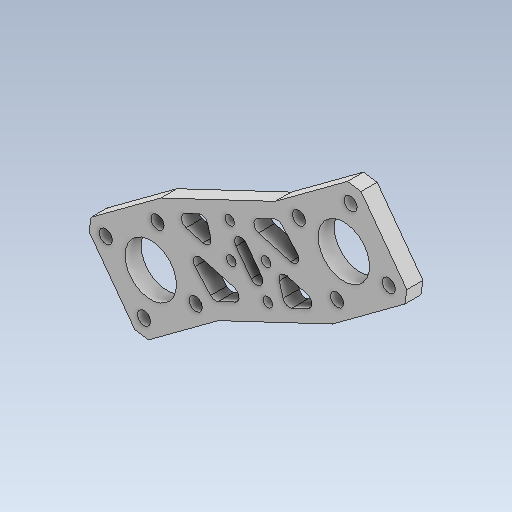
# Autodesk Inventor part: motor_holder_5
Saved by Autodesk Inventor 2020 (Build 240168000, 168)
## iProperties
Created: 2020-05-09
Part Number: motor_holder_5
Material: Generic
Document SubType Name: Modeling
Designer: psrobotics
Density: 1 g/cm^3
Appearance: Default
Author: psrobotics
Autodesk Inventor part; units mm, degrees
ref_plane "YZ Plane" through (0, 0, 0) normal (1, 0, 0) x (0, 1, 0)
ref_plane "XZ Plane" through (0, 0, 0) normal (0, 1, 0) x (-1, 0, 0)
ref_plane "XY Plane" through (0, 0, 0) normal (0, 0, 1) x (1, 0, 0)
sketch "Sketch1" plane through (0, 0, 0) normal (0, 0, 1) x (1, 0, 0)
  line L0 (79.7735, 25.7797) -> (84.0795, 21.6015) projected
  arc A0 (79.9013, 17.2954) -> (84.0795, 21.6015) centre (81.9904, 19.4484) ccw projected
  line L1 (79.9013, 17.2954) -> (75.5952, 21.4737) projected
  arc A1 (79.7735, 25.7797) -> (75.5952, 21.4737) centre (77.6844, 23.6267) ccw projected
  arc A2 (67.2283, 9.1476) -> (72.5711, 11.878) centre (69.8997, 10.5128) ccw projected
  line L2 (67.2283, 9.1476) -> (64.4979, 14.4903) projected
  arc A3 (69.8406, 17.2207) -> (64.4979, 14.4903) centre (67.1692, 15.8555) ccw projected
  line L3 (69.8406, 17.2207) -> (72.5711, 11.878) projected
  circle A4 centre (74.8858, 2.9538) radius 2.075 projected
  circle A5 centre (87.7531, 12.4634) radius 2.075 projected
  circle A6 centre (97.4816, -67.9698) radius 1.5 projected
  circle A7 centre (150.7021, -18.086) radius 1.5 projected
  circle A8 centre (148.9214, -29.9532) radius 1.5 projected
  circle A9 centre (85.6144, -66.1891) radius 1.5 projected
  arc A10 (80.4821, -2.1431) -> (77.7938, -6.6113) centre (99.1499, -16.4177) ccw projected
  arc A11 (83.0041, -2.3614) -> (80.4821, -2.1431) centre (81.6737, -3.0542) ccw projected
  line L4 (85.542, -7.2347) -> (83.0041, -2.3614) projected
  arc A12 (84.6624, -8.6966) -> (85.542, -7.2347) centre (84.655, -7.6966) ccw projected
  line L5 (79.168, -8.7372) -> (84.6624, -8.6966) projected
  arc A13 (77.7938, -6.6113) -> (79.168, -8.7372) centre (79.1569, -7.2373) ccw projected
  arc A14 (113.6374, -24.1387) -> (112.7579, -25.6006) centre (113.6448, -25.1387) ccw projected
  line L6 (119.1319, -24.0981) -> (113.6374, -24.1387) projected
  arc A15 (120.5061, -26.224) -> (119.1319, -24.0981) centre (119.1429, -25.5981) ccw projected
  arc A16 (117.8177, -30.6922) -> (120.5061, -26.224) centre (99.1499, -16.4177) ccw projected
  arc A17 (115.2958, -30.4739) -> (117.8177, -30.6922) centre (116.6262, -29.7811) ccw projected
  line L7 (112.7579, -25.6006) -> (115.2958, -30.4739) projected
  arc A18 (85.0937, -32.5635) -> (84.8754, -35.0855) centre (85.7865, -33.8939) ccw projected
  line L8 (89.967, -30.0256) -> (85.0937, -32.5635) projected
  arc A19 (91.4289, -30.9052) -> (89.967, -30.0256) centre (90.4289, -30.9125) ccw projected
  line L9 (91.4695, -36.3996) -> (91.4289, -30.9052) projected
  arc A20 (89.3436, -37.7738) -> (91.4695, -36.3996) centre (89.9695, -36.4107) ccw projected
  arc A21 (84.8754, -35.0855) -> (89.3436, -37.7738) centre (99.1499, -16.4177) ccw projected
  arc A22 (77.7938, -17.8952) -> (75.8562, -19.5241) centre (77.343, -19.3258) ccw projected
  line L10 (83.0344, -19.5466) -> (77.7938, -17.8952) projected
  arc A23 (83.4461, -21.2023) -> (83.0344, -19.5466) centre (82.7338, -20.5004) ccw projected
  line L11 (79.5897, -25.1161) -> (83.4461, -21.2023) projected
  arc A24 (77.1147, -24.5846) -> (79.5897, -25.1161) centre (78.5212, -24.0633) ccw projected
  arc A25 (75.8562, -19.5241) -> (77.1147, -24.5846) centre (99.1499, -16.4177) ccw projected
  arc A26 (122.4437, -13.3112) -> (121.1852, -8.2507) centre (99.1499, -16.4177) ccw projected
  arc A27 (120.506, -14.9401) -> (122.4437, -13.3112) centre (120.9569, -13.5095) ccw projected
  line L12 (115.2655, -13.2887) -> (120.506, -14.9401) projected
  arc A28 (114.8538, -11.6331) -> (115.2655, -13.2887) centre (115.5661, -12.3349) ccw projected
  line L13 (118.7102, -7.7192) -> (114.8538, -11.6331) projected
  arc A29 (121.1852, -8.2507) -> (118.7102, -7.7192) centre (119.7787, -8.772) ccw projected
  arc A30 (103.9345, -32.1215) -> (102.2789, -32.5332) centre (103.2327, -32.8338) ccw projected
  line L14 (107.8484, -35.9779) -> (103.9345, -32.1215) projected
  arc A31 (107.3169, -38.4529) -> (107.8484, -35.9779) centre (106.7956, -37.0464) ccw projected
  arc A32 (102.2564, -39.7114) -> (107.3169, -38.4529) centre (99.1499, -16.4177) ccw projected
  arc A33 (100.6275, -37.7738) -> (102.2564, -39.7114) centre (102.0581, -38.2246) ccw projected
  line L15 (102.2789, -32.5332) -> (100.6275, -37.7738) projected
  arc A34 (113.4245, 2.2501) -> (108.9563, 4.9385) centre (99.1499, -16.4177) ccw projected
  arc A35 (113.2062, -0.2718) -> (113.4245, 2.2501) centre (112.5134, 1.0586) ccw projected
  line L16 (108.3329, -2.8097) -> (113.2062, -0.2718) projected
  arc A36 (106.871, -1.9302) -> (108.3329, -2.8097) centre (107.871, -1.9228) ccw projected
  line L17 (106.8304, 3.5643) -> (106.871, -1.9302) projected
  arc A37 (108.9563, 4.9385) -> (106.8304, 3.5643) centre (108.3303, 3.5754) ccw projected
  line L18 (90.4515, 3.1426) -> (94.3653, -0.7138) projected
  arc A38 (90.983, 5.6176) -> (90.4515, 3.1426) centre (91.5043, 4.2111) ccw projected
  arc A39 (96.0435, 6.8761) -> (90.983, 5.6176) centre (99.1499, -16.4177) ccw projected
  arc A40 (97.6724, 4.9384) -> (96.0435, 6.8761) centre (96.2417, 5.3893) ccw projected
  line L19 (96.021, -0.3021) -> (97.6724, 4.9384) projected
  arc A41 (94.3653, -0.7138) -> (96.021, -0.3021) centre (95.0672, -0.0015) ccw projected
  circle A42 centre (111.213, -7.5024) radius 1.5 projected
  circle A43 centre (96.7757, -32.2405) radius 2 projected
  circle A44 centre (87.0868, -25.3329) radius 1.5 projected
  circle A45 centre (114.9728, -18.7919) radius 2 projected
  circle A46 centre (101.5242, -0.5948) radius 2 projected
  circle A47 centre (83.3271, -14.0434) radius 2 projected
  circle A48 centre (108.0652, -28.4808) radius 1.5 projected
  circle A49 centre (90.2347, -4.3545) radius 1.5 projected
  circle A50 centre (99.1499, -16.4177) radius 12 projected
  circle A51 centre (57.8427, 39.4747) radius 8 projected
  arc A52 (125.5376, -7.0532) -> (105.1801, 10.9253) centre (99.1499, -16.4177) ccw projected
  line L20 (105.1801, 10.9253) -> (80.5607, 34.8141) projected
  line L21 (80.5607, 34.8141) -> (61.3926, 60.7502) projected
  line L22 (36.4622, 42.3254) -> (61.3926, 60.7502) projected
  line L23 (36.4622, 42.3254) -> (55.6303, 16.3893) projected
  line L24 (55.6303, 16.3893) -> (71.2413, -14.1572) projected
  arc A53 (71.2413, -14.1572) -> (82.4532, -38.8947) centre (99.1499, -16.4177) ccw projected
  arc A54 (84.8089, -44.6016) -> (82.4532, -38.8947) centre (78.8753, -43.7112) ccw projected
  line L25 (84.8089, -44.6016) -> (81.0991, -69.3248) projected
  line L26 (81.0991, -69.3248) -> (100.8777, -72.2926) projected
  line L27 (100.8777, -72.2926) -> (104.5875, -47.5694) projected
  arc A55 (108.5144, -42.8053) -> (104.5875, -47.5694) centre (110.521, -48.4598) ccw projected
  arc A56 (108.5144, -42.8053) -> (121.627, -33.1144) centre (99.1499, -16.4177) ccw projected
  arc A57 (127.3339, -30.7587) -> (121.627, -33.1144) centre (126.4435, -36.6923) ccw projected
  line L28 (127.3339, -30.7587) -> (152.0571, -34.4685) projected
  line L29 (152.0571, -34.4685) -> (155.0249, -14.6899) projected
  line L30 (155.0249, -14.6899) -> (130.3017, -10.9801) projected
  arc A58 (125.5376, -7.0532) -> (130.3017, -10.9801) centre (131.1921, -5.0465) ccw projected
  line L31 (57.8427, 39.4747) -> (99.1499, -16.4177)
  line L32 (57.8427, 39.4747) -> (1.9503, -1.8326)
  line L33 (-1.5997, -23.1081) -> (-19.4302, 1.0181)
  line L34 (-19.4302, 1.0181) -> (61.3926, 60.7502)
  line L35 (61.3926, 60.7502) -> (79.2231, 36.624)
  line L36 (79.2231, 36.624) -> (-1.5997, -23.1081)
  line L37 (-1.5997, -23.1081) -> (61.3926, 60.7502) construction
  line L38 (-19.4302, 1.0181) -> (79.2231, 36.624) construction
  circle A59 centre (55.7441, 25.4892) radius 1.5 projected
  circle A60 centre (59.9412, 53.4603) radius 1.5 projected
  circle A61 centre (71.8282, 37.3762) radius 1.5 projected
  circle A62 centre (43.8571, 41.5733) radius 1.5 projected
  point P0 (0, 0)
  point P1 (29.8965, 18.8211)
  dimension "d0" = 69.5
  dimension "d1" = 30
  dimension "d2" = 100.5
  constraints: 16 end point, 3 midpoint, 3 perpendicular, 2 parallel
  measures "d0" distance of L31.start L32.end
  measures "d1" distance of L33.start L33.end
  measures "d2" distance of L33.end L34.end
extrude "Extrusion1" add sketch "Sketch1" along normal blind 5 contours L36 L23 L32 A51 L31 | L31 A51 L32 L23 L22 L21 L36 | L31 L32 A51 | A51 L32 L31 | L36 L33 L34 L23 | A59 | A60 | A61 | A62
sketch "Sketch2" plane through (0, 0, 5) normal (0, 0, 1) x (1, 0, 0)
  circle A0 centre (57.8427, 39.4747) radius 8 projected
  circle A1 centre (57.8427, 39.4747) radius 8
  point P0 (0, 0)
  dimension "d5" = 16
  constraints: 1 centre point, 1 coincident
  measures "d5" diameter of A1
extrude "Extrusion2" cut sketch "Sketch2" against normal blind 5
sketch "Sketch3" plane through (0, 0, 5) normal (0, 0, 1) x (1, 0, 0)
  circle A0 centre (57.8427, 39.4747) radius 8 projected
  line L0 (79.2231, 36.624) -> (61.3926, 60.7502) projected
  line L1 (61.3926, 60.7502) -> (-19.4302, 1.0181) projected
  line L2 (-19.4302, 1.0181) -> (-1.5997, -23.1081) projected
  line L3 (-1.5997, -23.1081) -> (79.2231, 36.624) projected
  line L4 (43.8571, 41.5733) -> (55.7441, 25.4892)
  line L5 (55.7441, 25.4892) -> (71.8282, 37.3762)
  line L6 (71.8282, 37.3762) -> (59.9412, 53.4603)
  line L7 (59.9412, 53.4603) -> (43.8571, 41.5733)
  line L8 (43.8571, 41.5733) -> (71.8282, 37.3762) construction
  line L9 (55.7441, 25.4892) -> (59.9412, 53.4603) construction
  point P0 (0, 0)
  dimension "d8" = 20
  dimension "d9" = 20
  constraints: 12 end point, 3 parallel, 2 midpoint, 1 perpendicular
  measures "d8" distance of L4.start L4.end
  measures "d9" distance of L5.end L4.end
hole "Hole1" at (43.8571, 41.5733, 5) at (59.9412, 53.4603, 5) at (71.8282, 37.3762, 5) at (55.7441, 25.4892, 5) direction (0, 0, -1) diameter 3 depth 17
sketch "Sketch10" plane through (0, 0, 5) normal (0, 0, 1) x (1, 0, 0)
  circle A0 centre (71.8282, 37.3762) radius 1.5 projected
  circle A1 centre (43.8571, 41.5733) radius 1.5 projected
  circle A2 centre (59.9412, 53.4603) radius 1.5 projected
  circle A3 centre (55.7441, 25.4892) radius 1.5 projected
  circle A4 centre (57.8427, 39.4747) radius 8 projected
  line L0 (-1.5997, -23.1081) -> (79.2231, 36.624) projected
  line L1 (79.2231, 36.624) -> (61.3926, 60.7502) projected
  line L2 (61.3926, 60.7502) -> (-19.4302, 1.0181) projected
  line L3 (-19.4302, 1.0181) -> (-1.5997, -23.1081) projected
  line L4 (36.4622, 42.3254) -> (54.2927, 18.1992) projected
  point P0 (0, 0)
extrude "Extrusion8" cut sketch "Sketch10" against normal blind 10 contours L3 L2 L4 L0
sketch "Sketch11" plane through (0, 0, 5) normal (0, 0, 1) x (1, 0, 0)
  circle A0 centre (-2.2147, 4.498) radius 4.075 projected
  line L0 (54.2927, 18.1992) -> (79.2231, 36.624) projected
  line L1 (36.4622, 42.3254) -> (54.2927, 18.1992) projected
  line L2 (0.9332, 25.4764) -> (18.7637, 1.3502)
  line L3 (18.7637, 1.3502) -> (-5.3625, -16.4803)
  line L4 (-5.3625, -16.4803) -> (-23.193, 7.6459)
  line L5 (-23.193, 7.6459) -> (0.9332, 25.4764)
  line L6 (0.9332, 25.4764) -> (-5.3625, -16.4803) construction
  line L7 (18.7637, 1.3502) -> (-23.193, 7.6459) construction
  line L8 (54.2927, 18.1992) -> (18.7637, 1.3502)
  line L9 (0.9332, 25.4764) -> (36.4622, 42.3254)
  point P0 (0, 0)
  dimension "d42" = 30
  dimension "d43" = 30
  constraints: 16 end point, 3 parallel, 2 midpoint, 1 perpendicular
  measures "d42" distance of L2.start L2.end
  measures "d43" distance of L2.end L3.end
extrude "Extrusion9" add sketch "Sketch11" against normal blind 5
sketch "Sketch12" plane through (0, 0, 5) normal (0, 0, 1) x (1, 0, 0)
  circle A0 centre (-2.2147, 4.498) radius 4.075 projected
  line L0 (54.2927, 18.1992) -> (79.2231, 36.624) projected
  line L1 (79.2231, 36.624) -> (61.3926, 60.7502) projected
  line L2 (61.3926, 60.7502) -> (36.4622, 42.3254) projected
  line L3 (36.4622, 42.3254) -> (0.9332, 25.4764) projected
  line L4 (0.9332, 25.4764) -> (-23.193, 7.6459) projected
  line L5 (-23.193, 7.6459) -> (-5.3625, -16.4803) projected
  line L6 (-5.3625, -16.4803) -> (18.7637, 1.3502) projected
  line L7 (18.7637, 1.3502) -> (54.2927, 18.1992) projected
  circle A1 centre (71.8282, 37.3762) radius 1.5 projected
  circle A2 centre (43.8571, 41.5733) radius 1.5 projected
  circle A3 centre (59.9412, 53.4603) radius 1.5 projected
  circle A4 centre (55.7441, 25.4892) radius 1.5 projected
  circle A5 centre (57.8427, 39.4747) radius 8 projected
  circle A6 centre (-2.2147, 4.498) radius 8
  line L8 (-0.1161, 18.4836) -> (-16.2002, 6.5966)
  line L9 (-16.2002, 6.5966) -> (-4.3132, -9.4875)
  line L10 (-4.3132, -9.4875) -> (11.7709, 2.3995)
  line L11 (11.7709, 2.3995) -> (-0.1161, 18.4836)
  line L12 (-0.1161, 18.4836) -> (-4.3132, -9.4875) construction
  line L13 (-16.2002, 6.5966) -> (11.7709, 2.3995) construction
  line L14 (-5.3625, -16.4803) -> (18.7637, 1.3502) projected
  circle A7 centre (11.7709, 2.3995) radius 1.5
  circle A8 centre (-4.3132, -9.4875) radius 1.5
  circle A9 centre (-16.2002, 6.5966) radius 1.5
  circle A10 centre (-0.1161, 18.4836) radius 1.5
  point P0 (0, 0)
  dimension "d46" = 16
  dimension "d47" = 20
  dimension "d48" = 20
  dimension "d49" = 3
  dimension "d50" = 3
  dimension "d51" = 3
  dimension "d52" = 3
  constraints: 12 end point, 5 centre point, 5 coincident, 3 parallel, 2 midpoint, 1 perpendicular
  measures "d46" diameter of A6
  measures "d47" distance of L8.start L8.end
  measures "d48" distance of L9.end L8.end
  measures "d49" diameter of A7
  measures "d50" diameter of A8
  measures "d51" diameter of A9
  measures "d52" diameter of A10
extrude "Extrusion10" cut sketch "Sketch12" against normal blind 5 contours A0 | A6 | L11 A10 L8 | L8 A10 L11 | A9 L9 L8 | L8 L9 A9 | A7 L10 L11 | L11 L10 A7 | A8 L10 L9 | L9 L10 A8
sketch "Sketch13" plane through (0, 0, 5) normal (0, 0, 1) x (1, 0, 0)
  circle A0 centre (-16.2002, 6.5966) radius 1.5 projected
  circle A1 centre (-0.1161, 18.4836) radius 1.5 projected
  circle A2 centre (-4.3132, -9.4875) radius 1.5 projected
  circle A3 centre (-2.2147, 4.498) radius 8 projected
  circle A4 centre (11.7709, 2.3995) radius 1.5 projected
  line L0 (54.2927, 18.1992) -> (79.2231, 36.624) projected
  line L1 (79.2231, 36.624) -> (61.3926, 60.7502) projected
  line L2 (61.3926, 60.7502) -> (36.4622, 42.3254) projected
  line L3 (36.4622, 42.3254) -> (0.9332, 25.4764) projected
  line L4 (0.9332, 25.4764) -> (-23.193, 7.6459) projected
  line L5 (-23.193, 7.6459) -> (-5.3625, -16.4803) projected
  line L6 (-5.3625, -16.4803) -> (18.7637, 1.3502) projected
  line L7 (18.7637, 1.3502) -> (54.2927, 18.1992) projected
  circle A5 centre (71.8282, 37.3762) radius 1.5 projected
  circle A6 centre (43.8571, 41.5733) radius 1.5 projected
  circle A7 centre (59.9412, 53.4603) radius 1.5 projected
  circle A8 centre (55.7441, 25.4892) radius 1.5 projected
  circle A9 centre (57.8427, 39.4747) radius 8 projected
  point P0 (0, 0)
hole "Hole3" at (71.8282, 37.3762, 5) at (55.7441, 25.4892, 5) at (43.8571, 41.5733, 5) at (59.9412, 53.4603, 5) at (11.7709, 2.3995, 5) at (-4.3132, -9.4875, 5) at (-0.1161, 18.4836, 5) at (-16.2002, 6.5966, 5) direction (0, 0, -1) diameter 4.1 depth 17
chamfer "Chamfer1" distance 3 angle 45 4 edges at (61.3926, 60.7502, 2.5) (79.2231, 36.624, 2.5) (-23.193, 7.6459, 2.5) (-5.3625, -16.4803, 2.5)
sketch "Sketch14" plane through (0, 0, 5) normal (0, 0, 1) x (1, 0, 0)
  line L0 (27.9353, 39.4155) -> (10.5493, 29.2901) projected
  line L1 (10.5493, 29.2901) -> (26.1882, 8.1293) projected
  line L2 (30.6819, 7.0022) -> (26.1882, 8.1293) projected
  line L3 (30.6819, 7.0022) -> (43.6756, 13.1643) projected
  line L4 (44.6032, 16.8624) -> (43.6756, 13.1643) projected
  line L5 (44.6032, 16.8624) -> (27.9353, 39.4155) projected
  circle A0 centre (33.6848, 24.7173) radius 1.5 projected
  circle A1 centre (22.8422, 19.5754) radius 1.5 projected
  circle A2 centre (34.207, 14.1043) radius 1.5 projected
  circle A3 centre (22.32, 30.1884) radius 1.5 projected
  point P0 (0, 0)
hole "Hole4" at (34.207, 14.1043, 5) at (33.6848, 24.7173, 5) at (22.8422, 19.5754, 5) at (22.32, 30.1884, 5) direction (0, 0, -1) diameter 3 depth 17
sketch "Sketch15" plane through (0, 0, 5) normal (0, 0, 1) x (1, 0, 0)
  circle A0 centre (22.8422, 19.5754) radius 1.5 projected
  circle A1 centre (34.207, 14.1043) radius 1.5 projected
  circle A2 centre (33.6848, 24.7173) radius 1.5 projected
  circle A3 centre (22.32, 30.1884) radius 1.5 projected
  line L0 (-2.9499, -14.6972) -> (-7.1456, -14.0677) projected
  line L1 (-2.9499, -14.6972) -> (18.7637, 1.3502) projected
  line L2 (18.7637, 1.3502) -> (54.2927, 18.1992) projected
  line L3 (54.2927, 18.1992) -> (76.8105, 34.841) projected
  line L4 (77.4401, 39.0367) -> (76.8105, 34.841) projected
  line L5 (77.4401, 39.0367) -> (63.1757, 58.3376) projected
  line L6 (58.98, 58.9672) -> (63.1757, 58.3376) projected
  line L7 (58.98, 58.9672) -> (36.4622, 42.3254) projected
  line L8 (36.4622, 42.3254) -> (0.9332, 25.4764) projected
  line L9 (0.9332, 25.4764) -> (-20.7804, 9.429) projected
  line L10 (-21.41, 5.2333) -> (-20.7804, 9.429) projected
  line L11 (-21.41, 5.2333) -> (-7.1456, -14.0677) projected
  circle A4 centre (-0.1161, 18.4836) radius 2.05 projected
  circle A5 centre (11.7709, 2.3995) radius 2.05 projected
  circle A6 centre (43.8571, 41.5733) radius 2.05 projected
  circle A7 centre (71.8282, 37.3762) radius 2.05 projected
  circle A8 centre (55.7441, 25.4892) radius 2.05 projected
  circle A9 centre (59.9412, 53.4603) radius 2.05 projected
  circle A10 centre (-4.3132, -9.4875) radius 2.05 projected
  circle A11 centre (-16.2002, 6.5966) radius 2.05 projected
  circle A12 centre (-2.2147, 4.498) radius 8 projected
  circle A13 centre (57.8427, 39.4747) radius 8 projected
  line L12 (3.5831, 22.8062) -> (14.8157, 28.133)
  line L13 (14.8157, 28.133) -> (17.4553, 18.979)
  line L14 (17.4553, 18.979) -> (3.5831, 22.8062)
  line L15 (6.9175, 17.4226) -> (28.9736, 11.3376)
  line L16 (28.9736, 11.3376) -> (17.4086, 5.8531)
  line L17 (17.4086, 5.8531) -> (6.9175, 17.4226)
  line L18 (36.4622, 42.3254) -> (0.9332, 25.4764) projected
  line L19 (39.5868, 15.1704) -> (36.7514, 25.0032)
  line L20 (36.7514, 25.0032) -> (51.6522, 20.8922)
  line L21 (51.6522, 20.8922) -> (39.5868, 15.1704)
  line L22 (37.5766, 38.1187) -> (47.9653, 26.662)
  line L23 (47.9653, 26.662) -> (26.1244, 32.6877)
  line L24 (26.1244, 32.6877) -> (37.5766, 38.1187)
  point P0 (0, 0)
  constraints: 24 end point, 10 parallel
extrude "Extrusion11" cut sketch "Sketch15" against normal blind 10 contours L12 L13 L14 | L15 L16 L17 | L19 L20 L21 | L22 L23 L24
fillet "Fillet1" radius 2 12 edges at (6.9175, 17.4226, 2.5) (28.9736, 11.3376, 2.5) (17.4086, 5.8531, 2.5) (17.4553, 18.979, 2.5) (3.5831, 22.8062, 2.5) (14.8157, 28.133, 2.5) (26.1244, 32.6877, 2.5) (37.5766, 38.1187, 2.5) (47.9653, 26.662, 2.5) (51.6522, 20.8922, 2.5) (36.7514, 25.0032, 2.5) (39.5868, 15.1704, 2.5)
sketch "Sketch16" plane through (0, 0, 5) normal (0, 0, 1) x (1, 0, 0)
  line L0 (41.3238, 28.4943) -> (31.3092, 31.2573) projected
  arc A0 (30.9841, 34.9923) -> (31.3092, 31.2573) centre (31.8411, 33.1852) ccw projected
  line L1 (30.9841, 34.9923) -> (36.2352, 37.4826) projected
  arc A1 (38.5738, 37.019) -> (36.2352, 37.4826) centre (37.0922, 35.6755) ccw projected
  line L2 (38.5738, 37.019) -> (43.3373, 31.7658) projected
  arc A2 (41.3238, 28.4943) -> (43.3373, 31.7658) centre (41.8557, 30.4223) ccw projected
  line L3 (13.559, 15.5903) -> (23.7888, 12.768) projected
  arc A3 (24.1139, 9.0329) -> (23.7888, 12.768) centre (23.2569, 10.84) ccw projected
  line L4 (24.1139, 9.0329) -> (18.7499, 6.4892) projected
  arc A4 (16.4114, 6.9528) -> (18.7499, 6.4892) centre (17.893, 8.2963) ccw projected
  line L5 (16.4114, 6.9528) -> (11.5455, 12.3189) projected
  arc A5 (13.559, 15.5903) -> (11.5455, 12.3189) centre (13.0271, 13.6623) ccw projected
  line L6 (46.7925, 18.5876) -> (41.7134, 16.1789) projected
  arc A6 (38.9347, 17.4319) -> (41.7134, 16.1789) centre (40.8564, 17.986) ccw projected
  line L7 (38.9347, 17.4319) -> (37.7411, 21.5711) projected
  arc A7 (40.1947, 24.0532) -> (37.7411, 21.5711) centre (39.6628, 22.1252) ccw projected
  line L8 (40.1947, 24.0532) -> (46.4674, 22.3226) projected
  arc A8 (46.7925, 18.5876) -> (46.4674, 22.3226) centre (45.9355, 20.3947) ccw projected
  line L9 (14.012, 19.9289) -> (8.7678, 21.3758) projected
  arc A9 (8.4428, 25.1108) -> (8.7678, 21.3758) centre (9.2998, 23.3037) ccw projected
  line L10 (8.4428, 25.1108) -> (12.6891, 27.1246) projected
  arc A10 (15.4678, 25.8716) -> (12.6891, 27.1246) centre (13.5461, 25.3175) ccw projected
  line L11 (15.4678, 25.8716) -> (16.4656, 22.411) projected
  arc A11 (14.012, 19.9289) -> (16.4656, 22.411) centre (14.5439, 21.8569) ccw projected
  circle A12 centre (22.8422, 19.5754) radius 1.5 projected
  circle A13 centre (34.207, 14.1043) radius 1.5 projected
  circle A14 centre (33.6848, 24.7173) radius 1.5 projected
  circle A15 centre (22.32, 30.1884) radius 1.5 projected
  line L12 (-2.9499, -14.6972) -> (-7.1456, -14.0677) projected
  line L13 (-2.9499, -14.6972) -> (18.7637, 1.3502) projected
  line L14 (18.7637, 1.3502) -> (54.2927, 18.1992) projected
  line L15 (54.2927, 18.1992) -> (76.8105, 34.841) projected
  line L16 (77.4401, 39.0367) -> (76.8105, 34.841) projected
  line L17 (77.4401, 39.0367) -> (63.1757, 58.3376) projected
  line L18 (58.98, 58.9672) -> (63.1757, 58.3376) projected
  line L19 (58.98, 58.9672) -> (36.4622, 42.3254) projected
  line L20 (36.4622, 42.3254) -> (0.9332, 25.4764) projected
  line L21 (0.9332, 25.4764) -> (-20.7804, 9.429) projected
  line L22 (-21.41, 5.2333) -> (-20.7804, 9.429) projected
  line L23 (-21.41, 5.2333) -> (-7.1456, -14.0677) projected
  circle A16 centre (-0.1161, 18.4836) radius 2.05 projected
  circle A17 centre (11.7709, 2.3995) radius 2.05 projected
  circle A18 centre (43.8571, 41.5733) radius 2.05 projected
  circle A19 centre (71.8282, 37.3762) radius 2.05 projected
  circle A20 centre (55.7441, 25.4892) radius 2.05 projected
  circle A21 centre (59.9412, 53.4603) radius 2.05 projected
  circle A22 centre (-4.3132, -9.4875) radius 2.05 projected
  circle A23 centre (-16.2002, 6.5966) radius 2.05 projected
  circle A24 centre (-2.2147, 4.498) radius 8 projected
  circle A25 centre (57.8427, 39.4747) radius 8 projected
  circle A26 centre (22.8422, 19.5754) radius 1.5 projected
  line L24 (22.8422, 19.5754) -> (33.6848, 24.7173)
  line L25 (34.207, 14.1043) -> (22.32, 30.1884)
  line L26 (25.8861, 25.3631) -> (30.6409, 18.9295) construction
  line L27 (24.2777, 24.1745) -> (29.0325, 17.7408)
  line L28 (32.2493, 20.1182) -> (27.4945, 26.5518)
  arc A27 (27.4945, 26.5518) -> (24.2777, 24.1745) centre (25.8861, 25.3631) ccw
  arc A28 (29.0325, 17.7408) -> (32.2493, 20.1182) centre (30.6409, 18.9295) ccw
  point P0 (0, 0)
  point P1 (28.2635, 22.1463)
  dimension "d75" = 4
  dimension "d76" = 4
  constraints: 12 end point, 4 point on circle, 4 tangent, 2 centre point, 2 midpoint, 1 parallel, 1 point on line
  measures "d75" distance of point (28.264, 22.146) L26.end
  measures "d76" diameter of A28
extrude "Extrusion12" cut sketch "Sketch16" against normal blind 10 contours L27 A27 L25 L24 | L24 L25 A28 L27 | L25 A27 L28 L24 | L24 L28 A28 L25
body "Solid1"
